Autodesk Fusion 360 part; units mm, degrees
note: some values were not read from the file. Chosen so that the rebuilt part matches the saved one: which face or edge a step refers to; which pieces of a blend or face edit are solid. Set by a fixed rule: which sketch regions a step uses.
(part 2 of 2)
mirror "Mirror1" about plane through (75.106127, 3.048, -98.051108) normal (1, 0, 0) of "Extrude6"
sketch "Sketch17" plane through (0, 6.096, 0) normal (0, 1, 0) x (-1, 0, 0)
  line L0 (-78.281127, -188.659261) -> (-78.281127, -194.86003)
  arc A0 (-86.145404, -193.998332) -> (-78.281127, -194.86003) centre (-74.930002, -127.95861) ccw
  line L1 (-86.145404, -193.998332) -> (-86.136723, -194.058614)
  line L2 (-86.079076, -194.458922) -> (-80.305461, -200.042609)
  arc A1 (-80.305461, -200.042609) -> (-69.916938, -200.068718) centre (-74.930002, -127.95861) ccw
  line L3 (-69.916938, -200.068718) -> (-64.140593, -194.510419)
  line L4 (-64.140593, -194.510419) -> (-64.07553, -194.058614)
  arc A2 (-71.931127, -194.876745) -> (-64.07553, -194.058614) centre (-74.930002, -127.95861) ccw
  line L5 (-71.931127, -194.876745) -> (-71.931127, -188.659261)
  arc A3 (-65.827056, -182.314025) -> (-71.931127, -188.659261) centre (-65.581127, -188.659261) ccw
  arc A4 (-65.827056, -182.314025) -> (-23.419721, -176.852239) centre (-75.106127, 57.096199) ccw
  arc A5 (-23.419721, -176.852239) -> (-8.849289, -154.51479) centre (-27.52935, -158.250803) ccw
  line L6 (-8.849289, -154.51479) -> (-11.007461, -143.72393)
  line L7 (-11.007461, -143.72393) -> (-8.36213, -140.0866)
  arc A6 (-3.039912, -139.24625) -> (-8.36213, -140.0866) centre (-5.280846, -142.327534) ccw
  line L8 (-3.039912, -139.24625) -> (9.700548, -148.512039)
  line L9 (12.339129, -150.464332) -> (16.304061, -138.860017)
  line L10 (16.304061, -138.860017) -> (16.137089, -138.78378)
  line L11 (16.137089, -138.78378) -> (11.088816, -140.667166)
  line L12 (11.088816, -140.667166) -> (11.019318, -140.819377)
  line L13 (11.019318, -140.819377) -> (1.075524, -133.587526)
  arc A7 (0.235173, -128.265308) -> (1.075524, -133.587526) centre (3.316458, -130.506242) ccw
  line L14 (0.235173, -128.265308) -> (6.995717, -118.96956)
  arc A8 (6.995717, -118.96956) -> (8.366095, -111.341172) centre (-0.193946, -113.740713) ccw
  line L15 (8.366095, -111.341172) -> (-23.189622, 1.229628)
  arc A9 (-16.660973, 0.953733) -> (-23.189622, 1.229628) centre (-19.910098, 1.451354) ccw
  arc A10 (-16.660973, 0.953733) -> (-10.384163, -0.007596) centre (-13.522568, 0.473068) ccw
  arc A11 (-10.384163, -0.007596) -> (-29.434159, -0.019779) centre (-19.910098, 1.451354) ccw
  line L16 (-29.434159, -0.019779) -> (2.25178, -113.05513)
  arc A12 (1.860243, -115.234669) -> (2.25178, -113.05513) centre (-0.193946, -113.740713) ccw
  line L17 (1.860243, -115.234669) -> (-17.125174, -141.339618)
  arc A13 (-17.125174, -141.339618) -> (-17.56166, -143.33171) centre (-15.070985, -142.833575) ccw
  line L18 (-17.56166, -143.33171) -> (-15.075976, -155.760128)
  arc A14 (-24.789597, -170.65176) -> (-15.075976, -155.760128) centre (-27.52935, -158.250803) ccw
  arc A15 (-125.422656, -170.65176) -> (-24.789597, -170.65176) centre (-75.106127, 57.096199) ccw
  arc A16 (-135.136278, -155.760128) -> (-125.422656, -170.65176) centre (-122.682903, -158.250803) ccw
  line L19 (-135.136278, -155.760128) -> (-132.650594, -143.33171)
  arc A17 (-132.650594, -143.33171) -> (-133.08708, -141.339618) centre (-135.141269, -142.833575) ccw
  line L20 (-133.08708, -141.339618) -> (-152.034083, -115.287488)
  arc A18 (-152.425798, -113.108587) -> (-152.034083, -115.287488) centre (-149.979894, -113.793532) ccw
  line L21 (-152.425798, -113.108587) -> (-151.469892, -109.695095)
  arc A19 (-151.469892, -109.695095) -> (-21.748345, -130.644222) centre (-45.713045, 133.067717) ccw
  arc A20 (-21.748345, -130.644222) -> (-22.481496, -123.208852) centre (-22.860001, -127.000004) ccw
  arc A21 (-143.161124, -90.146177) -> (-22.481496, -123.208852) centre (-28.068159, 93.172915) ccw
  arc A22 (-144.804126, -85.891994) -> (-143.161124, -90.146177) centre (-141.135269, -86.919412) ccw
  line L22 (-144.804126, -85.891994) -> (-120.850229, -0.353884)
  line L23 (-120.850229, -0.353884) -> (-120.778095, -0.019779)
  arc A23 (-120.778095, -0.019779) -> (-139.828091, -0.007596) centre (-130.302156, 1.451354) ccw
  arc A24 (-139.828091, -0.007596) -> (-133.55128, 0.953733) centre (-136.689686, 0.473068) ccw
  arc A25 (-127.031955, 1.119355) -> (-133.55128, 0.953733) centre (-130.302156, 1.451354) ccw
  line L24 (-127.031955, 1.119355) -> (-158.54056, -111.396223)
  arc A26 (-158.54056, -111.396223) -> (-157.169557, -119.022379) centre (-149.979894, -113.793532) ccw
  line L25 (-157.169557, -119.022379) -> (-150.447427, -128.265308)
  arc A27 (-151.287777, -133.587526) -> (-150.447427, -128.265308) centre (-153.528712, -130.506242) ccw
  line L26 (-151.287777, -133.587526) -> (-161.231572, -140.819377)
  line L27 (-161.231572, -140.819377) -> (-161.30107, -140.667166)
  line L28 (-161.30107, -140.667166) -> (-166.349343, -138.78378)
  line L29 (-166.349343, -138.78378) -> (-166.516315, -138.860017)
  line L30 (-166.516315, -138.860017) -> (-162.551383, -150.464332)
  line L31 (-159.912802, -148.512039) -> (-147.172342, -139.24625)
  arc A28 (-141.850124, -140.0866) -> (-147.172342, -139.24625) centre (-144.931408, -142.327534) ccw
  line L32 (-141.850124, -140.0866) -> (-139.204793, -143.72393)
  line L33 (-139.204793, -143.72393) -> (-141.362965, -154.51479)
  arc A29 (-141.362965, -154.51479) -> (-126.792533, -176.852239) centre (-122.682903, -158.250803) ccw
  arc A30 (-126.792533, -176.852239) -> (-84.385198, -182.314025) centre (-75.106127, 57.096199) ccw
  arc A31 (-78.281127, -188.659261) -> (-84.385198, -182.314025) centre (-84.631127, -188.659261) ccw
  line L34 (9.700548, -148.512039) -> (2.54, -157.480005)
  line L35 (2.54, -157.480005) -> (3.330318, -158.111041)
  line L36 (3.330318, -158.111041) -> (12.339129, -150.464332)
  line L37 (-162.551383, -150.464332) -> (-153.542572, -158.111041)
  line L38 (-153.542572, -158.111041) -> (-152.752254, -157.480005)
  line L39 (-152.752254, -157.480005) -> (-159.912802, -148.512039)
  line L40 (-86.136723, -194.058614) -> (-86.079076, -194.458922)
hidden bodies 1
